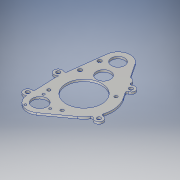
# Autodesk Inventor part: Motor Mount Plate
Saved by Autodesk Inventor 2019.4 (Build 234330000, 330)
## iProperties
Created: 2019-11-30
Part Number: Motor Mount Plate
Material: Aluminum 6061
Document SubType Name: Modeling
Designer: admin
Density: 2.7 g/cm^3
Appearance: Aluminum - Flat
Mass: 71.6386 g
Surface Area: 152.719 cm^2
Volume: 26.5328 cm^3
Author: admin
Autodesk Inventor part; units mm, degrees
ref_plane "YZ Plane" through (0, 0, 0) normal (1, 0, 0) x (0, 1, 0)
ref_plane "XZ Plane" through (0, 0, 0) normal (0, 1, 0) x (-1, 0, 0)
ref_plane "XY Plane" through (0, 0, 0) normal (0, 0, 1) x (1, 0, 0)
sketch "Sketch1" plane through (0, 0, 0) normal (0, 1, 0) x (-1, 0, 0)
  circle A0 centre (0, 0) radius 10
  circle A1 centre (11.9909, 79.0327) radius 10 construction
  circle A2 centre (11.9909, 79.0327) radius 10.5
  circle A3 centre (-8.6473, 36.4616) radius 22.3944 construction
  circle A4 centre (-8.6473, 36.4616) radius 25.3944
  circle A5 centre (6.4474, -27.1859) radius 9.5 projected
  arc A6 (1.4403, 93.6164) -> (29.9753, 79.7828) centre (11.9909, 79.0327) ccw construction
  arc A7 (-42.203, 13.9734) -> (31.4334, 31.4371) centre (-8.6473, 36.4616) ccw construction
  arc A8 (23.8115, -29.3627) -> (-8.0899, -36.9284) centre (6.4474, -27.1859) ccw construction
  line L0 (-8.0899, -36.9284) -> (-42.203, 13.9734)
  line L1 (23.8115, -29.3627) -> (31.4334, 31.4371)
  line L2 (-32.3242, 69.1894) -> (1.4403, 93.6164)
  line L3 (31.712, 38.145) -> (29.9753, 79.7828)
  arc A9 (29.9753, 79.7828) -> (1.4403, 93.6164) centre (11.9909, 79.0327) ccw
  arc A10 (-32.3242, 69.1894) -> (-42.203, 13.9734) centre (-8.6473, 36.4616) ccw
  arc A11 (31.712, 38.145) -> (-32.3242, 69.1894) centre (-8.6473, 36.4616) ccw construction
  arc A12 (31.4334, 31.4371) -> (31.712, 38.145) centre (-8.6473, 36.4616) ccw
  arc A13 (-8.0899, -36.9284) -> (23.8115, -29.3627) centre (6.4474, -27.1859) ccw
  dimension "d0" = 20
  dimension "d5" = 0.5
  dimension "d6" = 3
  dimension "d7" = 8
  dimension "d8" = 15
  dimension "d9" = 8
  constraints: 17 point on circle, 15 tangent, 11 centre point, 8 end point, 1 coincident
  measures "d0" diameter of A0
  measures "d5" radial gap between concentric circles of A1 A2
  measures "d6" radial gap between concentric circles of A3 A4
  measures "d7" radial gap between concentric circles of A1 A6
  measures "d8" radial gap between concentric circles of A4 A7
  measures "d9" radial gap between concentric circles of A5 A8
extrude "Extrusion1" add sketch "Sketch1" along normal blind 3
sketch "Sketch2" plane through (0, 0, 0) normal (0, -1, 0) x (1, 0, 0)
  circle A0 centre (35.2337, 17.429) radius 2.2
  circle A1 centre (-20.9595, 57.0259) radius 2.2
  circle A2 centre (13.6085, 72.7436) radius 2.2
  point P0 (0, 0)
  dimension "d12" = 4.4
  dimension "d13" = 4.4
  dimension "d14" = 4.4
  constraints: 3 centre point
  measures "d12" diameter of A0
  measures "d13" diameter of A2
  measures "d14" diameter of A1
extrude "Extrusion2" cut sketch "Sketch2" against normal blind 5
sketch "Sketch3" plane through (0, 0, 0) normal (0, -1, 0) x (1, 0, 0)
  circle A0 centre (35.893, -3.2614) radius 2.75
  circle A1 centre (35.893, -3.2614) radius 6
  circle A2 centre (49.8895, 56.3777) radius 2.75
  circle A3 centre (49.8895, 56.3777) radius 6
  circle A4 centre (-36.0964, 28.5483) radius 2.75
  circle A5 centre (-36.0964, 28.5483) radius 6
  circle A6 centre (-33.3464, 74.8865) radius 2.75
  circle A7 centre (-33.3464, 74.8865) radius 6
  point P0 (0, 0)
  dimension "d18" = 5.5
  dimension "d19" = 12
  dimension "d20" = 5.5
  dimension "d21" = 12
  dimension "d22" = 5.5
  dimension "d23" = 12
  dimension "d24" = 5.5
  dimension "d25" = 12
  constraints: 8 centre point, 4 coincident
  measures "d18" diameter of A0
  measures "d19" diameter of A1
  measures "d20" diameter of A2
  measures "d21" diameter of A3
  measures "d22" diameter of A4
  measures "d23" diameter of A5
  measures "d24" diameter of A6
  measures "d25" diameter of A7
extrude "Extrusion3" add sketch "Sketch3" against normal blind 3
fillet "Fillet1" radius 2 6 edges at (29.978, 1.5, -4.268) (34.5756, 1.5, 2.5922) (46.0191, 1.5, 51.793) (43.8922, 1.5, 56.1973) (-30.3974, 1.5, 69.6612) (-30.7339, 1.5, 25.857)
sketch "Sketch4" plane through (0, 0, 0) normal (0, -1, 0) x (1, 0, 0)
  circle A0 centre (23.213, -10.311) radius 2.413 projected
  circle A1 centre (-23.213, 10.311) radius 2.413 projected
  circle A2 centre (-20.5361, -14.9476) radius 2.413 projected
  circle A3 centre (23.213, -10.311) radius 2.75
  circle A4 centre (-23.213, 10.311) radius 2.75
  circle A5 centre (-20.5361, -14.9476) radius 2.75
  point P0 (0, 0)
  dimension "d29" = 5.5
  dimension "d30" = 5.5
  dimension "d31" = 5.5
  constraints: 3 centre point, 3 coincident
  measures "d29" diameter of A3
  measures "d30" diameter of A4
  measures "d31" diameter of A5
extrude "Extrusion4" cut sketch "Sketch4" against normal through all contours A0 | A1 | A2 | A3 | A4 | A5
sketch "Sketch5" plane through (0, 0, 0) normal (0, -1, 0) x (1, 0, 0)
  circle A0 centre (23.213, -10.311) radius 2.75 projected
  circle A1 centre (23.213, -10.311) radius 2.75
  circle A2 centre (23.213, -10.311) radius 6
  point P0 (0, 0)
  point P1 (25.9625, -10.2598)
  point P2 (24.2108, -12.8736)
  dimension "d34" = 12
  constraints: 2 coincident, 1 centre point, 3 other
  measures "d34" diameter of A2
extrude "Extrusion5" add sketch "Sketch5" against normal blind 3 contours A0 | A2
fillet "Fillet2" radius 2 2 edges at (28.1941, 1.5, -6.966) (21.9914, 1.5, -16.1853)
sketch "Sketch6" plane through (0, 3, 0) normal (0, 1, 0) x (1, 0, 0)
  circle A0 centre (-11.9909, -79.0327) radius 10.5 projected
  circle A1 centre (3.0091, -79.0327) radius 1.65
  line L0 (3.0091, -79.0327) -> (-11.9909, -79.0327) construction
  circle A2 centre (-19.4909, -66.0423) radius 1.65
  circle A3 centre (-19.4909, -92.023) radius 1.65
  point P0 (0, 0)
  dimension "d38" = 3.3
  dimension "d39" = 15
  dimension "d42" = 360
  constraints: 3 centre point, 2 end point, 1 horizontal, 7 other
  measures "d38" diameter of A1
  measures "d39" distance of L0.start L0.end
extrude "Extrusion6" cut sketch "Sketch6" against normal blind 10 contours A1 | A2 | A3
body "Solid1"
